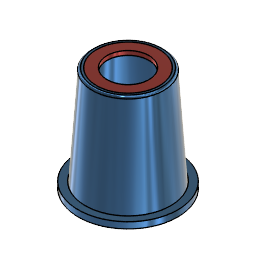
Collimator (Autodesk Fusion 360 design; units mm, degrees)
part number: 2026-01-28-17-58-51-538
Autodesk Fusion 360 part; units mm, degrees
sketch "Sketch1" plane through (0, 0, 0) normal (0, 1, 0) x (1, 0, 0)
  line L0 (-102, 0) -> (-85, -250)
  line L1 (-74.9769, -250) -> (-91.9769, 0)
  line L2 (-85, -250) -> (-74.9769, -250)
  line L3 (-102, 0) -> (-91.9769, 0)
  dimension "d2" = 102
  dimension "d4" = 10
  constraint parallel L0 L1
  constraint horizontal L2
  constraint parallel L2 L3
  measures "d2" distance of origin L0.start
  measures "d4" distance of L0 L1
revolve "Revolve1" add sketch "Sketch1" angle 360 about axis through (0, 0, 1.75) along (0, 0, 1) makes body 1
sketch "Sketch2" plane through (0, 0, 0) normal (0, 0, 1) x (1, 0, 0)
  circle A0 centre (0, 0) radius 75
  circle A1 centre (0, 0) radius 50
  dimension "d6" = 150
  dimension "d7" = 100
  constraint coincident A0.centre A1.centre
  constraint concentric A0 A1
  measures "d6" diameter of A0
  measures "d7" diameter of A1
extrude "Extrude1" add sketch "Sketch2" along normal blind 10 separate body makes body 2
move_body "Move1" bodies 2 to x (1, 0, 0) y (0, 1, 0) z (0, 0, 1) at (0, 0, 240)
sketch "Sketch3" plane through (0, 0, 0) normal (0, 0, 1) x (1, 0, 0)
fillet "Fillet1" radius 5 1 edges at (-79.2478, 30.7373, 250) on bodies 1
sketch "Sketch4" plane through (0, 0, 0) normal (0, 0, 1) x (1, 0, 0)
  circle A0 centre (0, 0) radius 119
  circle A1 centre (0, 0) radius 102
  dimension "d12" = 17
  constraint coincident A0.centre A1.centre
  measures "d12" distance of A0 A1
extrude "Extrude2" add sketch "Sketch4" along normal blind 15 separate body makes body 3
combine "Combine1" operation add target body 1 tool bodies 3
sketch "Sketch5" plane through (0, 0, 0) normal (0, 0, 1) x (1, 0, 0)
  circle A0 centre (0, 110) radius 3.8
  circle A1 centre (110, 0) radius 3.8
  circle A2 centre (-110, 0) radius 3.8
  circle A3 centre (0, -110) radius 3.8
  dimension "d15" = 7.6
  dimension "d16" = 7.6
  dimension "d17" = 7.6
  dimension "d18" = 7.6
  measures "d15" diameter of A0
  measures "d16" diameter of A1
  measures "d17" diameter of A2
  measures "d18" diameter of A3
extrude "Extrude3" cut sketch "Sketch5" along normal blind 8 bodies 1
